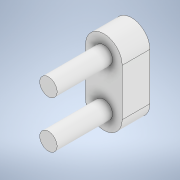
# Autodesk Inventor part: Pieza10
Saved by Autodesk Inventor 2022 (Build 260153000, 153)
## iProperties
Created: 2022-11-05
Part Number: Pieza10
Material: Resina acetálica, blanca
Document SubType Name: Modeling
Designer: Mauricio Guerrero
Density: 1.425 g/cm^3
Appearance: Suave - Blanco
Author: Mauricio Guerrero
Autodesk Inventor part; units mm, degrees
ref_plane "YZ Plane" through (0, 0, 0) normal (1, 0, 0) x (0, 1, 0)
ref_plane "XZ Plane" through (0, 0, 0) normal (0, 1, 0) x (-1, 0, 0)
ref_plane "XY Plane" through (0, 0, 0) normal (0, 0, 1) x (1, 0, 0)
sketch "Boceto1" plane through (0, 0, 0) normal (0, 0, 1) x (1, 0, 0)
  circle A0 centre (5.4445, 6.509) radius 1.25
  circle A1 centre (5.4445, -0.291) radius 1.25
  arc A2 (8.0824, 6.509) -> (2.8066, 6.509) centre (5.4445, 6.509) ccw
  arc A3 (2.8066, -0.291) -> (8.0824, -0.291) centre (5.4445, -0.291) ccw
  line L0 (2.8066, 6.509) -> (2.8066, -0.291)
  line L1 (8.0824, 6.509) -> (8.0824, -0.291)
  point P0 (0, 0)
  dimension "d0" = 2.5
  dimension "d1" = 2.5
  dimension "d6" = 2.6379
  dimension "d7" = 2.6379
  dimension "d8" = 6.8
  dimension "d9" = 5.2758
  constraints: 4 centre point, 4 end point, 4 point on circle, 2 coincident, 1 tangent, 1 vertical, 1 vertical alignment
  measures "d0" diameter of A0
  measures "d1" diameter of A1
  measures "d6" radius of A2
  measures "d7" radius of A3
  measures "d8" distance of L0.start L0.end
  measures "d9" distance between parallel lines of L1 L0
extrude "Extrusión1" add sketch "Boceto1" along normal blind 4
sketch "Boceto2" plane through (0, 0, 0) normal (0, 0, -1) x (-1, 0, 0)
  circle A0 centre (-5.4445, 6.509) radius 1.25 projected
  circle A1 centre (-5.4445, 6.509) radius 1.25
  circle A2 centre (-5.4445, -0.291) radius 1.25 projected
  circle A3 centre (-5.4445, -0.291) radius 1.25
  point P0 (0, 0)
  constraints: 2 centre point, 2 coincident
extrude "Extrusión2" add sketch "Boceto2" against normal blind 12
